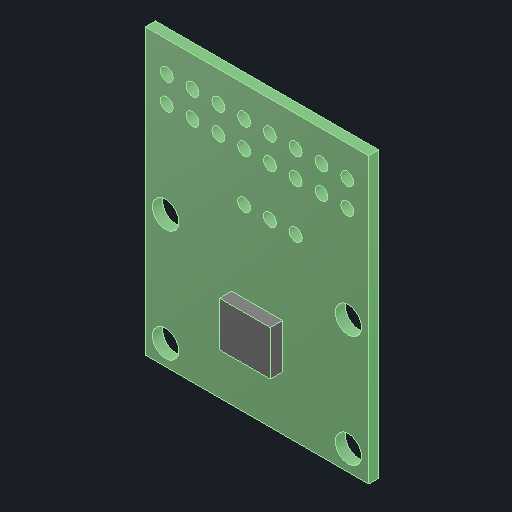
# Autodesk Inventor part: AS5047P-TS_EK_AB
Saved by Autodesk Inventor 2022 (Build 260153000, 153)
## iProperties
Created: 2021-07-13
Part Number: AS5047P-TS_EK_AB
Material: ABS プラスチック
Document SubType Name: Modeling
Designer: yuta0
Density: 1.06 g/cm^3
Appearance: 滑らか - 濃い深緑
Description: 在庫有
購入先: Digikey
在庫数: 6.0
Author: yuta0
Autodesk Inventor part; units mm, degrees
ref_plane "YZ Plane" through (0, 0, 0) normal (1, 0, 0) x (0, 1, 0)
ref_plane "XZ Plane" through (0, 0, 0) normal (0, 1, 0) x (-1, 0, 0)
ref_plane "XY Plane" through (0, 0, 0) normal (0, 0, 1) x (1, 0, 0)
sketch "スケッチ1" plane through (0, 0, 0) normal (0, 0, 1) x (1, 0, 0)
  line L0 (-11, -7.5) -> (11, -7.5)
  line L1 (11, -7.5) -> (11, 20.5)
  line L2 (11, 20.5) -> (-11, 20.5)
  line L3 (-11, 20.5) -> (-11, -7.5)
  line L4 (-11, -7.5) -> (11, 20.5) construction
  line L5 (11, -7.5) -> (-11, 20.5) construction
  line L6 (-9, -5.5) -> (9, -5.5) construction
  line L7 (9, -5.5) -> (9, 5.5) construction
  line L8 (9, 5.5) -> (-9, 5.5) construction
  line L9 (-9, 5.5) -> (-9, -5.5) construction
  line L10 (-9, -5.5) -> (9, 5.5) construction
  line L11 (9, -5.5) -> (-9, 5.5) construction
  point P0 (0, 0)
  point P1 (0, 6.5)
  point P2 (0, 6.5)
  point P3 (0, 0)
  point P4 (0, 0)
  point P5 (0, 0)
  dimension "d0" = 22
  dimension "d1" = 28
  dimension "d2" = 18
  dimension "d3" = 11
  dimension "d4" = 2
  constraints: 24 end point, 7 midpoint, 4 parallel, 2 coincident, 2 horizontal, 2 perpendicular, 1 vertical alignment
  measures "d0" distance of L0.start L0.end
  measures "d1" distance of L0.end L1.end
  measures "d2" distance of L7.end L8.end
  measures "d3" distance of L6.end L7.end
  measures "d4" distance between parallel lines of L0 L6
extrude "押し出し1" add sketch "スケッチ1" against normal blind 1
sketch "スケッチ2" plane through (0, 0, 0) normal (0, 0, 1) x (1, 0, 0)
  line L0 (-9, -5.5) -> (9, -5.5)
  line L1 (9, -5.5) -> (9, 5.5)
  line L2 (9, 5.5) -> (-9, 5.5)
  line L3 (-9, 5.5) -> (-9, -5.5)
  line L4 (-9, -5.5) -> (9, 5.5) construction
  line L5 (9, -5.5) -> (-9, 5.5) construction
  point P0 (0, 0)
  dimension "d7" = 11
  dimension "d8" = 18
  constraints: 12 end point, 2 midpoint, 2 parallel, 1 horizontal, 1 perpendicular
  measures "d7" distance of L0.end L1.end
  measures "d8" distance of L1.end L2.end
hole "穴1" at (-9, 5.5, 0) at (-9, -5.5, 0) at (9, 5.5, 0) at (9, -5.5, 0) direction (0, 0, -1) diameter 2.6 end through all
sketch "スケッチ3" plane through (0, 0, 0) normal (0, 0, 1) x (1, 0, 0)
  line L0 (-2.5, -2.2) -> (2.5, -2.2)
  line L1 (2.5, -2.2) -> (2.5, 2.2)
  line L2 (2.5, 2.2) -> (-2.5, 2.2)
  line L3 (-2.5, 2.2) -> (-2.5, -2.2)
  line L4 (-2.5, -2.2) -> (2.5, 2.2) construction
  line L5 (2.5, -2.2) -> (-2.5, 2.2) construction
  point P0 (0, 0)
  dimension "d16" = 4.4
  dimension "d17" = 5
  constraints: 12 end point, 2 midpoint, 2 parallel, 1 horizontal, 1 perpendicular
  measures "d16" distance of L0.end L1.end
  measures "d17" distance of L1.end L2.end
extrude "押し出し2" add sketch "スケッチ3" along normal blind 1.2
sketch "スケッチ4" plane through (0, 0, 0) normal (0, 0, 1) x (1, 0, 0)
  line L0 (-11, 20.5) -> (-11, -7.5) projected
  line L1 (-11, 20.5) -> (11.0137, 20.4892) construction
  line L2 (11.0137, 20.4892) -> (11, -7.5) construction
  line L3 (11, -7.5) -> (-11.0137, -7.4892) construction
  line L4 (-11.0137, -7.4892) -> (-11, 20.5) construction
  line L5 (11, -7.5) -> (11, 20.5) projected
  line L6 (-11, -7.5) -> (11, -7.5) projected
  circle A0 centre (-1.27, 17.4952) radius 0.635
  circle A1 centre (1.27, 17.494) radius 0.635
  circle A2 centre (-1.27, 14.9552) radius 0.635
  circle A3 centre (1.27, 14.954) radius 0.635
  circle A4 centre (-3.81, 14.9565) radius 0.635
  circle A5 centre (-3.81, 17.4965) radius 0.635
  circle A6 centre (-6.35, 14.9577) radius 0.635
  circle A7 centre (-6.35, 17.4977) radius 0.635
  circle A8 centre (-8.89, 14.959) radius 0.635
  circle A9 centre (-8.89, 17.499) radius 0.635
  circle A10 centre (3.81, 17.4928) radius 0.635
  circle A11 centre (3.81, 14.9528) radius 0.635
  circle A12 centre (6.35, 17.4915) radius 0.635
  circle A13 centre (6.35, 14.9515) radius 0.635
  circle A14 centre (8.89, 17.4903) radius 0.635
  circle A15 centre (8.89, 14.9503) radius 0.635
  circle A16 centre (-1.27, 10.1952) radius 0.635
  circle A17 centre (1.27, 10.194) radius 0.635
  circle A18 centre (3.81, 10.1928) radius 0.635
  point P0 (0, 0)
  dimension "d25" = 3
  dimension "d30" = 2.54
  dimension "d32" = 1.27
  dimension "d37" = 1.27
  dimension "d38" = 1.27
  dimension "d39" = 3
  dimension "d41" = 2.54
  dimension "d43" = 2.54
  dimension "d45" = 1.27
  dimension "d46" = 1.27
  dimension "d53" = 2.54
  dimension "d63" = 2.54
  dimension "d71" = 1.27
  dimension "d73" = 10.3
  dimension "d78" = 2.54
  constraints: 19 centre point, 3 vertical alignment, 2 point on line, 33 other
  measures "d25" distance from line of L1 A0.centre
  measures "d30" distance of A1.centre A0.centre
  measures "d32" horizontal distance of point (0, 0) A0.centre
  measures "d37" diameter of A0
  measures "d38" diameter of A1
  measures "d39" distance from line of L1 A1.centre
  measures "d41" distance of A0.centre A2.centre
  measures "d43" distance of A3.centre A1.centre
  measures "d45" diameter of A2
  measures "d46" diameter of A3
  measures "d53" distance of A2.centre A4.centre
  measures "d63" distance of A1.centre A10.centre
  measures "d71" diameter of A16
  measures "d73" distance from line of L1 A16.centre
  measures "d78" distance of A16.centre A17.centre
extrude "押し出し3" cut sketch "スケッチ4" against normal through all
equation "\"d45\" = d37"
equation "\"d46\" = d45"
equation "\"d71\" = d45"
